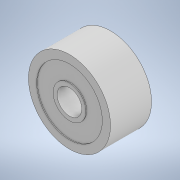
# Autodesk Inventor part: bearing_3_10_5
Saved by Autodesk Inventor 2020 (Build 240168000, 168)
## iProperties
Created: 2019-05-09
Part Number: bearing_3_10_5
Material: Generic
Document SubType Name: Modeling
Designer: psrob
Density: 1 g/cm^3
Appearance: Default
Author: psrob
Autodesk Inventor part; units mm, degrees
ref_plane "YZ Plane" through (0, 0, 0) normal (1, 0, 0) x (0, 1, 0)
ref_plane "XZ Plane" through (0, 0, 0) normal (0, 1, 0) x (-1, 0, 0)
ref_plane "XY Plane" through (0, 0, 0) normal (0, 0, 1) x (1, 0, 0)
sketch "Sketch1" plane through (0, 0, 0) normal (0, 0, 1) x (1, 0, 0)
  circle A0 centre (14.3651, 1.9735) radius 1.5 projected
  circle A1 centre (14.3651, 1.9735) radius 5
  circle A2 centre (14.3651, 1.9735) radius 1.5
  point P0 (0, 0)
  dimension "d0" = 10
  dimension "d1" = 3
  constraints: 2 centre point, 2 coincident
  measures "d0" diameter of A1
  measures "d1" diameter of A2
extrude "Extrusion1" add sketch "Sketch1" along normal blind 5
sketch "Sketch2" plane through (14.3651, 1.9735, 5) normal (0, 0, 1) x (1, 0, 0)
  circle A0 centre (0, 0) radius 5 projected
  circle A1 centre (0, 0) radius 1.5 projected
  circle A2 centre (0, 0) radius 2
  circle A3 centre (0, 0) radius 4
  point P0 (-14.3651, -1.9735)
  dimension "d4" = 4
  dimension "d5" = 8
  constraints: 2 centre point, 2 coincident
  measures "d4" diameter of A2
  measures "d5" diameter of A3
extrude "Extrusion2" cut sketch "Sketch2" against normal blind 0.1 contours A3
sketch "Sketch3" plane through (14.3651, 1.9735, 0) normal (0, 0, -1) x (-1, 0, 0)
  circle A0 centre (0, 0) radius 4 projected
  circle A1 centre (0, 0) radius 2 projected
  point P0 (14.3651, -1.9735)
extrude "Extrusion3" cut sketch "Sketch3" against normal blind 0.1
body "Solid1"
